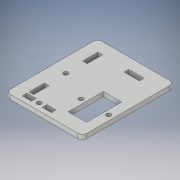
# Autodesk Inventor part: 板子1
Saved by Autodesk Inventor 2017 (Build 210142000, 142)
## iProperties
Part Number: 板子1
Material: 一般
Document SubType Name: Modeling
Designer: User
Density: 1 g/cm^3
Appearance: 預設
Author: User
Autodesk Inventor part; units mm, degrees
ref_plane "YZ Plane" through (0, 0, 0) normal (1, 0, 0) x (0, 1, 0)
ref_plane "XZ Plane" through (0, 0, 0) normal (0, 1, 0) x (-1, 0, 0)
ref_plane "XY Plane" through (0, 0, 0) normal (0, 0, 1) x (1, 0, 0)
sketch "草圖1" plane through (0, 0, 0) normal (0, 1, 0) x (-1, 0, 0)
  line L0 (-25, 27) -> (-25, -27)
  line L1 (-25, -30) -> (24.1827, -30)
  line L2 (17.3, 27) -> (11.3, 27)
  line L3 (11.3, 27) -> (11.3, 24)
  line L4 (11.3, 24) -> (17.3, 24)
  line L5 (17.3, 24) -> (17.3, 27)
  line L6 (17.3, 22.5) -> (14.3, 22.5)
  line L7 (14.3, 22.5) -> (14.3, 12.5)
  line L8 (14.3, 12.5) -> (17.3, 12.5)
  line L9 (17.3, 12.5) -> (17.3, 22.5)
  line L10 (14.3, 12.5) -> (15.8, 12.5)
  circle A0 centre (15.8, 0) radius 1.5
  line L11 (14.3, -22.5) -> (17.3, -22.5)
  line L12 (17.3, -22.5) -> (17.3, -12.5)
  line L13 (17.3, -12.5) -> (14.3, -12.5)
  line L14 (14.3, -12.5) -> (14.3, -22.5)
  circle A1 centre (7.8, 25.5) radius 1.5
  line L15 (-1.7, 24) -> (4.3, 24)
  line L16 (4.3, 24) -> (4.3, 27)
  line L17 (4.3, 27) -> (-1.7, 27)
  line L18 (-1.7, 27) -> (-1.7, 24)
  line L19 (-6.7, 21) -> (-18.7, 21)
  line L20 (-18.7, 21) -> (-18.7, -2)
  line L21 (-18.7, -2) -> (-6.7, -2)
  line L22 (-6.7, -2) -> (-6.7, 21)
  line L23 (-6.7, 21) -> (-6.7, 9.5)
  circle A2 centre (-3.7, 9.5) radius 1.5
  circle A3 centre (-21.7, 9.5) radius 1.5
  line L24 (-2.5, -19.8) -> (-12.5, -19.8)
  line L25 (-12.5, -19.8) -> (-12.5, -22.8)
  line L26 (-12.5, -22.8) -> (-2.5, -22.8)
  line L27 (-2.5, -22.8) -> (-2.5, -19.8)
  line L28 (-25, -30) -> (-25, -27)
  line L29 (-12.5, -22.8) -> (-12.5, -21.3)
  line L30 (25, 30) -> (25, -30)
  line L31 (25, -30) -> (24.1827, -30)
  line L32 (25, 30) -> (25, 27)
  line L33 (-25, 30) -> (-25, 27)
  line L34 (0, -42) -> (0, 42) projected
  line L35 (35, 0) -> (-35, 0) projected
  line L36 (25, 30) -> (25, 27)
  line L37 (25, 30) -> (-25, 30)
  point P0 (25, -30)
  dimension "d1" = 50
  dimension "d46" = 3
  dimension "d47" = 1.5
  dimension "d48" = 3
  dimension "d49" = 10
  dimension "d50" = 3
  dimension "d51" = 1.5
  dimension "d53" = 3
  dimension "d54" = 3
  dimension "d55" = 10
  dimension "d56" = 3
  dimension "d61" = 3
  dimension "d62" = 6
  dimension "d63" = 3
  dimension "d67" = 12
  dimension "d68" = 23
  dimension "d69" = 11.5
  dimension "d72" = 3
  dimension "d73" = 3
  dimension "d74" = 10
  dimension "d75" = 3
  dimension "d88" = 60
  dimension "d91" = 25
  dimension "d92" = 30
  constraints: 72 end point, 8 perpendicular, 6 parallel, 6 point on line, 4 centre point, 3 midpoint, 2 collinear, 1 horizontal, 1 vertical
  measures "d1" distance of L30.start L33.start
  measures "d46" distance of L4.end L5.end
  measures "d47" distance of L4.end L6.start
  measures "d48" distance of L6.start L6.end
  measures "d49" distance of L6.end L10.start
  measures "d50" distance of L10.start L9.start
  measures "d51" distance of L10.start L10.end
  measures "d53" diameter of A0
  measures "d54" distance of L13.start L13.end
  measures "d55" distance of L13.end L14.end
  measures "d56" distance of L14.end L12.start
  measures "d61" diameter of A1
  measures "d62" distance of L18.end L15.end
  measures "d63" distance of L15.end L17.start
  measures "d67" distance of L22.end L20.start
  measures "d68" distance of L20.start L20.end
  measures "d69" distance of L22.end L23.end
  measures "d72" diameter of A2
  measures "d73" diameter of A3
  measures "d74" distance of L27.end L24.end
  measures "d75" distance of L27.start L27.end
  measures "d88" distance of L30.start L30.end
  measures "d91" distance between parallel lines of L34 L30
  measures "d92" distance between parallel lines of L35 L1
extrude "擠出2" add sketch "草圖1" along normal mid plane 3 contours L33 L37 L34 L17 L18 L15 L35 L22 L19 L20 L0 | L35 L20 L21 L22 L34 L1 L28 L0 | L37 L30 L35 A0 L34 L15 L16 L17 | L34 L35 A0 L30 L31 L1
fillet "圓角1" radius 3 4 edges at (-25, 0, 30) (25, 0, 30) (-25, 0, -30) (25, 0, -30)
